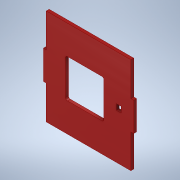
# Autodesk Inventor part: Part3
Saved by Autodesk Inventor 2020 (Build 240168000, 168)
## iProperties
Created: 2020-03-09
Part Number: Part3
Material: Generic
Document SubType Name: Modeling
Designer: tor16003
Density: 1 g/cm^3
Appearance: Red
Author: tor16003
Autodesk Inventor part; units mm, degrees
ref_plane "YZ Plane" through (0, 0, 0) normal (1, 0, 0) x (0, 1, 0)
ref_plane "XZ Plane" through (0, 0, 0) normal (0, 1, 0) x (-1, 0, 0)
ref_plane "XY Plane" through (0, 0, 0) normal (0, 0, 1) x (1, 0, 0)
sketch "Sketch1" plane through (0, 0, 0) normal (0, 0, 1) x (1, 0, 0)
  line L0 (-3, 35) -> (0, 35)
  line L1 (-3, 35) -> (-3, 65)
  line L2 (-3, 65) -> (0, 65)
  line L3 (0, 65) -> (0, 100)
  line L4 (0, 100) -> (88, 100)
  line L5 (88, 100) -> (88, 65)
  line L6 (88, 65) -> (91, 65)
  line L7 (91, 65) -> (91, 35)
  line L8 (91, 35) -> (88, 35)
  line L9 (88, 35) -> (88, 0)
  line L10 (88, 0) -> (0, 0)
  line L11 (0, 0) -> (0, 35)
  line L12 (78, 53) -> (73, 53)
  line L13 (73, 53) -> (73, 47)
  line L14 (73, 47) -> (78, 47)
  line L15 (78, 47) -> (78, 53)
  point P0 (78, 50)
  point P1 (91, 50)
  dimension "d0" = 3
  dimension "d10" = 30
  dimension "d21" = 35
  dimension "d22" = 100
  dimension "d23" = 5
  dimension "d24" = 6
  dimension "d30" = 88
  dimension "d31" = 10
  dimension "d32" = 3
  constraints: 32 end point, 8 perpendicular, 4 horizontal, 4 parallel, 2 collinear, 2 midpoint, 1 coincident, 1 horizontal alignment, 1 vertical
  measures "d0" distance of L0.start L0.end
  measures "d10" distance of L6.end L7.end
  measures "d21" distance of L8.end L9.end
  measures "d22" distance of L9.end L4.end
  measures "d23" distance of L14.end L13.end
  measures "d24" distance of L12.end L13.end
  measures "d30" distance between parallel lines of L11 L9
  measures "d31" distance between parallel lines of L5 L15
  measures "d32" distance between parallel lines of L5 L7
extrude "Extrusion1" add sketch "Sketch1" along normal blind 3
sketch "Boceto2" plane through (0, 0, 3) normal (0, 0, 1) x (1, 0, 0)
  line L0 (58, 70) -> (22, 70)
  line L1 (20, 68) -> (20, 32)
  line L2 (22, 30) -> (58, 30)
  line L3 (60, 32) -> (60, 68)
  line L4 (88, 100) -> (0, 100) projected
  line L5 (0, 100) -> (0, 65) projected
  arc A0 (60, 68) -> (58, 70) centre (58, 68) ccw
  arc A1 (58, 30) -> (60, 32) centre (58, 32) ccw
  arc A2 (22, 70) -> (20, 68) centre (22, 68) ccw
  arc A3 (20, 32) -> (22, 30) centre (22, 32) ccw
  point P0 (0, 0)
  dimension "d33" = 40
  dimension "d34" = 40
  dimension "d35" = 30
  dimension "d36" = 20
  dimension "d37" = 2
  constraints: 8 end point, 8 point on circle, 8 tangent, 4 centre point, 3 equal radius, 2 parallel, 1 horizontal, 1 perpendicular
  measures "d33" distance between parallel lines of L1 L3
  measures "d34" distance between parallel lines of L2 L0
  measures "d35" distance between parallel lines of L4 L0
  measures "d36" distance between parallel lines of L5 L1
  measures "d37" radius of A0
extrude "Extrusión2" cut sketch "Boceto2" against normal blind 3
body "Solid1"
